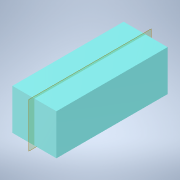
# Autodesk Inventor part: Contenedor B
Saved by Autodesk Inventor 2020.3 (Build 243373000, 373)
## iProperties
Created: 2020-07-23
Part Number: Contenedor B
Material: ABS Plastic
Document SubType Name: Modeling
Designer: juanp
Density: 1.06 g/cm^3
Appearance: Smooth - White
Mass: 373.524 g
Surface Area: 1735.81 cm^2
Volume: 352.381 cm^3
Author: juanp
Autodesk Inventor part; units mm, degrees
ref_plane "YZ Plane" through (0, 0, 0) normal (1, 0, 0) x (0, 1, 0)
ref_plane "XZ Plane" through (0, 0, 0) normal (0, 1, 0) x (-1, 0, 0)
ref_plane "XY Plane" through (0, 0, 0) normal (0, 0, 1) x (1, 0, 0)
sketch "Sketch1" plane through (0, 0, 0) normal (0, 1, 0) x (-1, 0, 0)
  line L0 (0, 0) -> (-80, 0)
  line L1 (-80, 0) -> (-80, -202)
  line L2 (-80, -202) -> (0, -202)
  line L3 (0, -202) -> (0, 0)
  line L4 (-4, -4) -> (-38, -4)
  line L5 (-38, -4) -> (-38, -39.6)
  line L6 (-38, -39.6) -> (-4, -39.6)
  line L7 (-4, -39.6) -> (-4, -4)
  line L8 (-4, -43.6) -> (-38, -43.6)
  line L9 (-38, -43.6) -> (-38, -79.2)
  line L10 (-38, -79.2) -> (-4, -79.2)
  line L11 (-4, -79.2) -> (-4, -43.6)
  line L12 (-4, -83.2) -> (-38, -83.2)
  line L13 (-38, -83.2) -> (-38, -118.8)
  line L14 (-38, -118.8) -> (-4, -118.8)
  line L15 (-4, -118.8) -> (-4, -83.2)
  line L16 (-4, -122.8) -> (-38, -122.8)
  line L17 (-38, -122.8) -> (-38, -158.4)
  line L18 (-38, -158.4) -> (-4, -158.4)
  line L19 (-4, -158.4) -> (-4, -122.8)
  line L20 (-4, -162.4) -> (-38, -162.4)
  line L21 (-38, -162.4) -> (-38, -198)
  line L22 (-38, -198) -> (-4, -198)
  line L23 (-4, -198) -> (-4, -162.4)
  line L24 (-76, -198) -> (-42, -198)
  line L25 (-42, -162.4) -> (-76, -162.4)
  line L26 (-42, -198) -> (-42, -162.4)
  line L27 (-76, -162.4) -> (-76, -198)
  line L28 (-76, -158.4) -> (-42, -158.4)
  line L29 (-76, -122.8) -> (-76, -158.4)
  line L30 (-42, -122.8) -> (-76, -122.8)
  line L31 (-42, -158.4) -> (-42, -122.8)
  line L32 (-76, -118.8) -> (-42, -118.8)
  line L33 (-76, -83.2) -> (-76, -118.8)
  line L34 (-42, -118.8) -> (-42, -83.2)
  line L35 (-42, -4) -> (-76, -4)
  line L36 (-76, -4) -> (-76, -39.6)
  line L37 (-76, -39.6) -> (-42, -39.6)
  line L38 (-42, -83.2) -> (-76, -83.2)
  line L39 (-76, -79.2) -> (-42, -79.2)
  line L40 (-42, -43.6) -> (-76, -43.6)
  line L41 (-76, -43.6) -> (-76, -79.2)
  line L42 (-42, -79.2) -> (-42, -43.6)
  line L43 (-42, -39.6) -> (-42, -4)
  dimension "d0" = 34
  dimension "d1" = 35.6
  dimension "d2" = 4
  dimension "d3" = 4
  dimension "d6" = 39.6
  dimension "d11" = 4
  dimension "d14" = 38
  dimension "d19" = 4
  constraints: 88 end point, 4 parallel, 3 horizontal, 2 perpendicular, 1 vertical, 72 other
  measures "d0" distance of L6.end L5.end
  measures "d1" distance of L5.end L4.end
  measures "d2" distance between parallel lines of L0 L4
  measures "d3" distance between parallel lines of L3 L7
  measures "d6" distance of L4.start L8.start
  measures "d11" distance between parallel lines of L2 L22
  measures "d14" distance of L22.end L24.end
  measures "d19" distance between parallel lines of L1 L27
extrude "Extrusion1" add sketch "Sketch1" along normal blind 70
sketch "Sketch2" plane through (0, 70, 0) normal (0, 1, 0) x (1, 0, 0)
  line L0 (0, 0) -> (80, 0) projected
  line L1 (0, 202) -> (0, 0) projected
  line L2 (80, 0) -> (80, 202) projected
  line L3 (80, 202) -> (0, 202) projected
extrude "Extrusion2" add sketch "Sketch2" along normal blind 4
ref_plane "Work Plane4" through (40, 0, -202) normal (-1, 0, 0) x (0, 0, 1)
fillet "Fillet1" radius 15 40 edges at (21, 70, -198) (4, 70, -180.2) (59, 70, -198) (42, 70, -180.2) (59, 70, -158.4) (42, 70, -140.6) (21, 70, -158.4) (4, 70, -140.6) (59, 70, -118.8) (42, 70, -101) (21, 70, -118.8) (4, 70, -101) (21, 70, -79.2) (4, 70, -61.4) (59, 70, -79.2) (42, 70, -61.4) (59, 70, -39.6) (42, 70, -21.8) (21, 70, -39.6) (4, 70, -21.8) (76, 70, -21.8) (59, 70, -4) (38, 70, -21.8) (21, 70, -4) (38, 70, -61.4) (21, 70, -43.6) (76, 70, -61.4) (59, 70, -43.6) (76, 70, -101) (59, 70, -83.2) (76, 70, -140.6) (59, 70, -122.8) (38, 70, -140.6) (21, 70, -122.8) (38, 70, -180.2) (21, 70, -162.4) (76, 70, -180.2) (59, 70, -162.4) (38, 70, -101) (21, 70, -83.2)
body "Solid1"
